Autodesk Fusion 360 part; units mm, degrees
(part 2 of 2)
equation "material_thickness = 4 mm"
equation "nut_width = 3 mm"
equation "nut_height = 1.2 mm"
equation "screw_length = 6.1 mm"
equation "screw_hole_diameter = 1.6 mm"
equation "d358 = object_height + 2 * tolerance_to_object"
equation "d361 = object_length / 2 + tolerance_to_object"
equation "d368 = d19 - pin_thickness"
equation "d385 = pin_thickness"
equation "d386 = pin_thickness"
equation "d387 = d386"
equation "d388 = pin_thickness"
equation "d389 = d388"
equation "d391 = pin_thickness"
equation "d392 = pin_thickness"
equation "d394 = d395"
equation "d395 = pin_thickness"
equation "d396 = d397"
equation "d397 = pin_thickness"
equation "d399 = pin_thickness"
equation "d401 = -d361"
equation "d402 = screw_hole_diameter"
equation "d403 = screw_hole_diameter"
equation "d404 = screw_hole_diameter"
equation "d405 = screw_hole_diameter"
equation "d406 = nut_width"
equation "d407 = nut_height"
equation "d409 = screw_hole_diameter"
equation "d410 = screw_hole_diameter"
equation "d411 = nut_width"
equation "d413 = nut_height"
equation "d420 = screw_length"
equation "d421 = material_thickness"
equation "d422 = material_thickness"
equation "d424 = screw_length"
equation "d425 = material_thickness"
equation "d426 = material_thickness"
equation "d427 = pin_thickness"
equation "d428 = pin_thickness"
equation "d429 = pin_thickness"
equation "d430 = pin_thickness"
equation "d433 = d428"
equation "d434 = d430"
equation "d435 = screw_hole_diameter"
equation "d436 = screw_hole_diameter"
equation "d437 = d399"
equation "d438 = d385"
equation "d439 = d391"
equation "d440 = d392"
equation "d441 = -material_thickness"
equation "d443 = material_thickness"
equation "d445 = material_thickness"
equation "d448 = -material_thickness"
equation "d450 = -object_width / 2 - tolerance_to_object"
equation "d451 = object_width / 2 + tolerance_to_object"
equation "d452 = nut_height"
equation "d453 = nut_width"
equation "d454 = screw_hole_diameter"
equation "d455 = screw_length"
equation "d456 = nut_width"
equation "d457 = screw_hole_diameter"
equation "d458 = nut_height"
equation "d459 = screw_length"
equation "d460 = screw_hole_diameter"
equation "d461 = nut_width"
equation "d462 = nut_height"
equation "d463 = screw_length"
equation "d464 = nut_height"
equation "d465 = screw_hole_diameter"
equation "d466 = nut_width"
equation "d467 = screw_length"
equation "d468 = material_thickness"
equation "d470 = -material_thickness"
equation "mid_layer_spacing = ( object_height + 2 * tolerance_to_object ) - 16 mm - tolerance_to_object"
equation "d473 = mid_layer_spacing"
equation "d474 = pin_thickness"
equation "d475 = pin_thickness"
equation "d476 = pin_thickness"
equation "d477 = pin_thickness"
equation "d478 = material_thickness"
equation "d480 = material_thickness"
equation "d482 = d427"
equation "d483 = d429"
equation "pin_rail_length = 45.84 mm"
equation "pin_rail_width = 2.52 mm"
equation "d489 = pin_rail_width"
equation "d490 = pin_rail_length"
equation "d491 = tolerance_to_object"
equation "d492 = pin_rail_width"
equation "d493 = pin_rail_length"
equation "d494 = tolerance_to_object"
equation "pin_rail_distance_to_back = 2.98 mm"
equation "d496 = pin_rail_distance_to_back"
equation "d497 = pin_rail_distance_to_back"
equation "jst_connector_width = 7.80 mm"
equation "jst_connector_length = 14.00 mm"
equation "d500 = jst_connector_width"
equation "d501 = jst_connector_length"
equation "d508 = 2 * tolerance_to_object"
equation "d509 = 2 * tolerance_to_object"
equation "d510 = 2 * tolerance_to_object"
equation "d513 = tolerance_to_object * 2"
